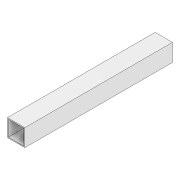
# Autodesk Inventor part: Cablecanal Ranurado 30x30 L=255 mm
Saved by Autodesk Inventor 2020 (Build 240168000, 168)
## iProperties
Created: 2020-07-11
Part Number: Cablecanal Ranurado 30x30 L=255 mm
Material: PPS Plastic
Document SubType Name: Modeling
Designer: Hernan
Density: 1.637 g/cm^3
Appearance: Smooth - White
Author: Hernan
Autodesk Inventor part; units mm, degrees
ref_plane "YZ Plane" through (0, 0, 0) normal (1, 0, 0) x (0, 1, 0)
ref_plane "XZ Plane" through (0, 0, 0) normal (0, 1, 0) x (-1, 0, 0)
ref_plane "XY Plane" through (0, 0, 0) normal (0, 0, 1) x (1, 0, 0)
sketch "Sketch1" plane through (0, 0, 0) normal (0, 0, 1) x (1, 0, 0)
  line L0 (-17.2121, 7.0196) -> (12.7879, 7.0196)
  line L1 (12.7879, 7.0196) -> (12.7879, -22.9804)
  line L2 (12.7879, -22.9804) -> (-17.2121, -22.9804)
  line L3 (-17.2121, -22.9804) -> (-17.2121, 7.0196)
  line L4 (11.0879, -22.9804) -> (11.0879, 7.0196)
  line L5 (-17.2121, 5.3196) -> (12.7879, 5.3196)
  line L6 (-15.5121, 7.0196) -> (-15.5121, -22.9804)
  line L7 (-17.2121, -21.2804) -> (12.7879, -21.2804)
  point P0 (-15.5121, -21.2804)
  point P1 (11.0879, -21.2804)
  point P2 (11.0879, 5.3196)
  point P3 (-15.5121, 5.3196)
  dimension "d1" = 30
  dimension "d2" = 30
  dimension "d3" = 1.7
  dimension "d4" = 1.7
  dimension "d5" = 1.7
  dimension "d6" = 1.7
  constraints: 16 end point, 8 point on line, 3 horizontal, 2 parallel, 2 vertical, 1 perpendicular
  measures "d1" distance of L0.start L0.end
  measures "d2" distance of L0.end L1.end
  measures "d3" distance between parallel lines of L0 L5
  measures "d4" distance between parallel lines of L3 L6
  measures "d5" distance between parallel lines of L2 L7
  measures "d6" distance between parallel lines of L1 L4
extrude "Extrusion1" add sketch "Sketch1" against normal blind 255
extrude "Extrusion2" cut sketch "Sketch1" against normal blind 430 contours L5 L4 L7 L6
body "Solid1"
